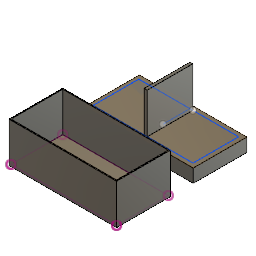
magnetidea v1 (Autodesk Fusion 360 design; units mm, degrees)
Autodesk Fusion 360 part; units mm, degrees
box "BoxPrimitive1" add length 50.8 width 101.6 height 38.1 placed x (0, 0, 1) y (1, 0, 0) z (0, 1, 0) at (0, 0, 0) makes body 1
shell "Shell1" thickness 1 removed faces 1 at (33.8667, 38.1, 16.9333) on bodies 1
sketch "Sketch2" plane through (0, 1, 0) normal (0, 1, 0) x (-1, 0, 0)
  line L0 (-1, 49.8) -> (-100.6, 49.8)
  line L1 (-100.6, 49.8) -> (-100.6, 1)
  line L2 (-100.6, 1) -> (-1, 1)
  line L3 (-1, 1) -> (-1, 49.8)
sketch "Sketch3" plane through (0, 1, 0) normal (0, 1, 0) x (-1, 0, 0)
  line L0 (-1, 49.8) -> (-1, 1)
  line L1 (-100.6, 49.8) -> (-100.6, 1)
  line L2 (-1, 49.8) -> (-100.6, 49.8)
  line L3 (-100.6, 49.8) -> (-1, 49.8)
  line L4 (-1, 1) -> (-100.6, 1)
box "BoxPrimitive3" add length 50.8 width 101.6 height 12.7 placed x (0, 0, 1) y (1, 0, 0) z (0, 1, 0) at (1, 1, -71.3648) separate body makes body 2
sketch "Sketch4" plane through (0, 13.7, 0) normal (0, 1, 0) x (-1, 0, 0)
  line L0 (-1, -20.5648) -> (-102.6, -20.5648)
  line L1 (-102.6, -20.5648) -> (-102.6, -71.3648)
  line L2 (-102.6, -71.3648) -> (-1, -71.3648)
  line L3 (-1, -71.3648) -> (-1, -20.5648)
  line L4 (-4.2209, -67.5341) -> (-52.4809, -67.5341)
  line L5 (-52.4809, -67.5341) -> (-52.4809, -42.1341)
  line L6 (-55.3, -67.5341) -> (-98.48, -67.5341)
  line L7 (-4.2209, -67.5341) -> (-98.48, -67.5341)
  line L8 (-98.48, -67.5341) -> (-98.48, -24.4733)
  line L9 (-98.48, -24.4733) -> (-4.2209, -24.4733)
  line L10 (-4.2209, -24.4733) -> (-4.2209, -67.5341)
  dimension "d20" = 48.26
  dimension "d21" = 25.4
  dimension "d22" = 43.18
  measures "d20" distance of origin
box "BoxPrimitive4" add length 43.0608 width 2.819 height 38.1 placed x (0, 0, 1) y (1, 0, 0) z (0, 1, 0) at (52.4809, 13.7, -67.5341) bodies 2
